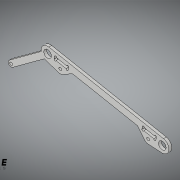
# Autodesk Inventor part: 台形サスバー
Saved by Autodesk Inventor 2019 (Build 230136000, 136)
## iProperties
Created: 2019-09-17
Part Number: 台形サスバー
Material: 一般
Document SubType Name: Modeling
Designer: tanjihayato
Density: 1 g/cm^3
Appearance: 既定
Author: tanjihayato
Autodesk Inventor part; units mm, degrees
ref_plane "YZ Plane" through (0, 0, 0) normal (1, 0, 0) x (0, 1, 0)
ref_plane "XZ Plane" through (0, 0, 0) normal (0, 1, 0) x (-1, 0, 0)
ref_plane "XY Plane" through (0, 0, 0) normal (0, 0, 1) x (1, 0, 0)
sketch "スケッチ2" plane through (0, 0, 0) normal (0, 0, 1) x (1, 0, 0)
  circle A0 centre (127.6431, 30.2622) radius 1.5
  circle A1 centre (5.9362, 53.5882) radius 1.5
  line L0 (5.9362, 53.5882) -> (127.6431, 30.2622) construction
  circle A2 centre (5.9362, 53.5882) radius 4.025
  circle A3 centre (127.6431, 30.2622) radius 4.025
  arc A4 (127.2517, 23.2481) -> (128.9655, 37.1616) centre (127.6431, 30.2622) ccw
  line L1 (12.8357, 52.2659) -> (13.4004, 55.2122)
  line L2 (15.4628, 54.817) -> (26.0698, 52.7841)
  line L3 (28.1322, 52.3888) -> (27.5675, 49.4424)
  line L4 (14.8981, 51.8706) -> (25.5051, 49.8377)
  line L5 (120.7437, 31.5845) -> (121.3084, 34.5309)
  line L6 (119.246, 34.9262) -> (108.639, 36.9591)
  line L7 (106.5765, 37.3543) -> (106.0119, 34.408)
  line L8 (108.0743, 34.0127) -> (118.6813, 31.9798)
  circle A5 centre (19.3546, 46.4346) radius 3
  circle A6 centre (112.5307, 28.5767) radius 3
  line L9 (7.2586, 60.4876) -> (128.9655, 37.1616)
  arc A7 (17.9263, 42.1672) -> (21.5465, 42.5045) centre (19.3546, 46.4346) ccw
  arc A8 (109.041, 25.7356) -> (112.28, 24.0837) centre (112.5307, 28.5767) ccw
  line L10 (3.7066, 46.9264) -> (17.9263, 42.1672)
  line L11 (112.28, 24.0837) -> (127.2517, 23.2481)
  circle A9 centre (19.3546, 46.4346) radius 1.5
  circle A10 centre (112.5307, 28.5767) radius 1.5
  line L12 (32.3442, 48.5269) -> (21.5465, 42.5045)
  line L13 (109.041, 25.7356) -> (101.2351, 35.3235)
  line L14 (32.3442, 48.5269) -> (101.2351, 35.3235)
  arc A11 (108.639, 36.9591) -> (106.5765, 37.3543) centre (107.6078, 37.1567) ccw
  arc A12 (106.0119, 34.408) -> (108.0743, 34.0127) centre (107.0431, 34.2103) ccw
  arc A13 (121.3084, 34.5309) -> (119.246, 34.9262) centre (120.2772, 34.7285) ccw
  arc A14 (118.6813, 31.9798) -> (120.7437, 31.5845) centre (119.7125, 31.7821) ccw
  arc A15 (28.1322, 52.3888) -> (26.0698, 52.7841) centre (27.101, 52.5864) ccw
  arc A16 (25.5051, 49.8377) -> (27.5675, 49.4424) centre (26.5363, 49.64) ccw
  arc A17 (15.4628, 54.817) -> (13.4004, 55.2122) centre (14.4316, 55.0146) ccw
  arc A18 (12.8357, 52.2659) -> (14.8981, 51.8706) centre (13.8669, 52.0682) ccw
  line L15 (5.9362, 53.5882) -> (-32.8159, 25.1361) construction
  circle A19 centre (-32.8159, 25.1361) radius 1.5
  arc A20 (-34.5914, 27.5543) -> (-31.0404, 22.7179) centre (-32.8159, 25.1361) ccw
  line L16 (-34.5914, 27.5543) -> (-0.9595, 52.247)
  line L17 (-31.0404, 22.7179) -> (2.5914, 47.4106)
  arc A21 (7.2586, 60.4876) -> (-0.9595, 52.247) centre (5.9362, 53.5882) ccw
  arc A22 (2.5914, 47.4106) -> (3.7066, 46.9264) centre (5.9362, 53.5882) ccw
  point P0 (0, 0)
  point P1 (0, 0)
  dimension "d31" = 8.05
  dimension "d32" = 8.05
  dimension "d33" = 3
  dimension "d34" = 3
  dimension "d35" = 15
  dimension "d36" = 3
  dimension "d37" = 15
  dimension "d38" = 6
  dimension "d39" = 6
  dimension "d40" = 9
  dimension "d41" = 9
  dimension "d42" = 3
  dimension "d43" = 3
  dimension "d44" = 7.5
  dimension "d45" = 7.5
  dimension "d46" = 40
  dimension "d47" = 40
  dimension "d48" = 2.1
  dimension "d49" = 2.1
  dimension "d50" = 2.1
  dimension "d51" = 2.1
  dimension "d52" = 2.1
  dimension "d53" = 2.1
  dimension "d54" = 2.1
  dimension "d55" = 2.1
  dimension "d56" = 3
  dimension "d57" = 6
  dimension "d58" = 3
  dimension "d59" = 3
  constraints: 36 end point, 28 point on circle, 23 centre point, 22 tangent, 14 point on line, 8 coincident, 4 parallel, 4 perpendicular, 1 collinear
  measures "d31" diameter of A2
  measures "d32" diameter of A3
  measures "d33" radial gap between concentric circles of A3 A4
  measures "d34" distance of L1.start L1.end
  measures "d35" distance of L1.end L3.start
  measures "d36" distance of L5.start L5.end
  measures "d37" distance of L5.end L7.start
  measures "d38" diameter of A5
  measures "d39" diameter of A6
  measures "d40" diameter of A7
  measures "d41" diameter of A8
  measures "d42" diameter of A9
  measures "d43" diameter of A10
  measures "d44" distance from line of A5.centre L3
  measures "d45" distance from line of A10.centre L7
  measures "d46" angle of L13 L0
  measures "d47" angle of L0 L12
  measures "d48" diameter of A11
  measures "d49" diameter of A12
  measures "d50" diameter of A13
  measures "d51" diameter of A14
  measures "d52" diameter of A15
  measures "d53" diameter of A16
  measures "d54" diameter of A17
  measures "d55" diameter of A18
  measures "d56" diameter of A19
  measures "d57" diameter of A20
  measures "d58" radial gap between concentric circles of A21 A2
  measures "d59" radial gap between concentric circles of A22 A2
extrude "押し出し2" add sketch "スケッチ2" along normal blind 3 contours L11 A8 L13 L14 L12 A7 L10 A22 L17 A20 L16 A21 L9 A4 | A5 | A6
equation "\"d47\" = d46"
